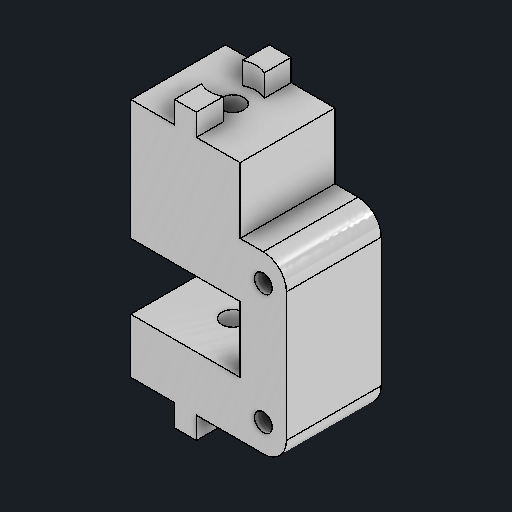
# Autodesk Inventor part: B Idler (Tulip)
Saved by Autodesk Inventor 2026.2 (Build 302298000, 298)
## iProperties
Created: 2025-04-15
Part Number: B Idler (Tulip)
Material: Aluminum 6061
Document SubType Name: Modeling
Designer: Joshua Eah
Density: 2.7 g/cm^3
Appearance: Machined - Aluminum
Author: Joshua Eah
Autodesk Inventor part; units mm, degrees
ref_plane "YZ Plane" through (0, 0, 0) normal (1, 0, 0) x (0, 1, 0)
ref_plane "XZ Plane" through (0, 0, 0) normal (0, 1, 0) x (-1, 0, 0)
sketch "Base Profile" plane through (0, 0, 0) normal (0, 1, 0) x (-1, 0, 0)
  line L0 (0, 0) -> (-15, 0)
  line L1 (-15, 0) -> (-15, -13)
  line L2 (-15, -13) -> (0, -13)
  line L3 (0, -13) -> (0, 0)
  line L4 (-15, -13) -> (-21.35, -13)
  line L5 (-21.35, -13) -> (-21.35, 0)
  line L6 (-21.35, 0) -> (-15, 0)
  line L7 (-7.5, -13) -> (-7.5, 0) construction
  circle A0 centre (-7.5, -6.5) radius 1.5
  line L8 (-6, -13) -> (-6, 0)
  line L9 (-9, -13) -> (-9, 0)
  circle A1 centre (-7.5, -6.5) radius 3.175
  point P0 (-9, 0)
  dimension "d376" = 15
  dimension "d380" = 13
  dimension "d381" = 6.35
  dimension "d395" = 3
  dimension "d405" = 6.35
  constraints: 20 end point, 4 perpendicular, 3 midpoint, 2 centre point, 2 coincident, 2 horizontal, 2 parallel, 2 point on line, 2 symmetric about line, 1 tangent
  measures "d376" distance of L2.end L1.end
  measures "d380" distance of L4.end L5.end
  measures "d381" distance between parallel lines of L5 L1
  measures "d395" diameter of A0
  measures "d405" diameter of A1
extrude "Stock" add sketch "Base Profile" along normal blind 33
ref_plane "Work Plane3" through (0, 16.5, 0) normal (0, -1, 0) x (1, 0, 0)
extrude "Guide" add sketch "Base Profile" against normal blind 3 contours L8 A1 L9 L0 | L8 A0 L9 A1 | L2 L9 A1 L8 | A0 | L8 A1 L9 A0
mirror "Mirror3" about plane through (0, 16.5, 0) normal (0, -1, 0) of "Guide"
sketch "Front Profile" plane through (0, 0, 0) normal (0, 0, 1) x (1, 0, 0)
  line L0 (21.35, 0) -> (21.35, 33) projected
  line L1 (0, 33) -> (6, 33) projected
  line L2 (0, 0) -> (0, 33) projected
  line L3 (0, 16.5) -> (21.35, 16.5)
  line L4 (0, 7.5) -> (21.35, 7.5)
  line L5 (15, 33) -> (15, 0)
  line L6 (9, 0) -> (21.35, 0) projected
  line L7 (0, 0) -> (6, 0) projected
  line L8 (6, 0) -> (6, -3) projected
  line L9 (9, -3) -> (6, -3) projected
  line L10 (9, 0) -> (9, -3) projected
  line L11 (9, 33) -> (21.35, 33) projected
  line L12 (9, 33) -> (9, 36) projected
  line L13 (9, 36) -> (6, 36) projected
  line L14 (6, 33) -> (6, 36) projected
  line L15 (15, 24) -> (21.35, 24)
  line L16 (15, 16.5) -> (21.35, 24) construction
  line L17 (21.35, 7.5) -> (15, 0) construction
  circle A0 centre (18.175, 20.25) radius 1.5
  circle A1 centre (18.175, 3.75) radius 1.5
  point P0 (15, 7.5)
  dimension "d383" = 9
  dimension "d384" = 6.35
  dimension "d408" = 7.5
  dimension "d409" = 7.5
  dimension "d413" = 3
  dimension "d414" = 3
  constraints: 12 end point, 5 midpoint, 5 point on line, 3 perpendicular, 2 centre point, 1 parallel
  measures "d383" distance between parallel lines of L3 L4
  measures "d384" distance between parallel lines of L0 L5
  measures "d408" distance between parallel lines of L4 L6
  measures "d409" distance between parallel lines of L15 L3
  measures "d413" diameter of A0
  measures "d414" diameter of A1
extrude "Bearing Clearance" cut sketch "Front Profile" against normal through all contours L4 L2 L3 L5
extrude "Hole Clearance" cut sketch "Base Profile" against normal blind 3 from surface at 36 contours A1 L8 | L8 A0 L9 A1 | L9 A1 | A0 | L8 A1 L9 A0
hole "Hole25" at (7.5, 0, -6.5) direction (0, 1, 0) diameter 3 end through all
extrude "Extrusion22" cut sketch "Front Profile" against normal through all contours L15 L5 L11 L0
fillet "Fillet3" radius 3.175 2 edges at (21.35, 24, -6.5) (21.35, 0, -6.5)
hole "Hole26" at (18.175, 20.25, 0) at (18.175, 3.75, 0) direction (0, 0, -1) diameter 2.459 end through all thread size "M3x0.5" class "6H" standard "ANSI Metric M Profile"
equation "\"extrusionWidth\" = 15"
equation "\"idlerLength\" = 0"
equation "\"bearingOffsetFromBottom\" = 7.5"
equation "\"extrusionOffset\" = 33"
equation "\"d165\" = extrusionWidth"
equation "\"bearingStackHeight\" = 9"
equation "\"bearingSlotLength\" = 0"
equation "\"bearingClearance\" = 13"
equation "\"pinSupportLength\" = 2"
body "Solid3"
